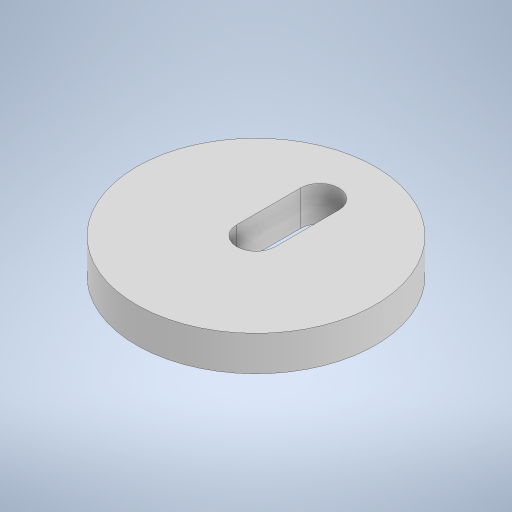
# Autodesk Inventor part: M3_15_ホーン
Saved by Autodesk Inventor 2024.1 (Build 281209000, 209)
## iProperties
Created: 2024-04-01
Part Number: M3_15_ホーン
Material: 一般
Document SubType Name: Modeling
Designer: hibik
Density: 1 g/cm^3
Appearance: 既定
Author: hibik
Autodesk Inventor part; units mm, degrees
ref_plane "YZ Plane" through (0, 0, 0) normal (1, 0, 0) x (0, 1, 0)
ref_plane "XZ Plane" through (0, 0, 0) normal (0, 1, 0) x (-1, 0, 0)
ref_plane "XY Plane" through (0, 0, 0) normal (0, 0, 1) x (1, 0, 0)
sketch "スケッチ1" plane through (0, 0, 0) normal (0, 1, 0) x (-1, 0, 0)
  circle A0 centre (0, 0) radius 22.5 construction
  circle A1 centre (0, 0) radius 25.5 construction
  line L0 (25.5, 1.2181) -> (25.5, -1.2181)
  line L1 (25.5, 1.2181) -> (22.3764, 2.355)
  line L2 (25.5, -1.2181) -> (22.3764, -2.355)
  line L3 (35.7, 0) -> (-35.7, 0) projected
  circle A2 centre (0, 0) radius 18.75
  line L4 (22.3764, -2.355) -> (18.647, -1.9625)
  line L5 (22.3764, 2.355) -> (18.647, 1.9625)
  line L6 (19.484, 11.2527) -> (16.2367, 9.3773)
  line L7 (22.8, 11.4846) -> (19.484, 11.2527)
  line L8 (22.8, 11.4846) -> (23.7909, 9.259)
  line L9 (23.7909, 9.259) -> (21.3997, 6.9499)
  line L10 (21.3997, 6.9499) -> (17.8331, 5.7916)
  line L11 (13.2226, 18.2047) -> (11.0189, 15.1706)
  line L12 (16.1576, 19.7653) -> (13.2226, 18.2047)
  line L13 (16.1576, 19.7653) -> (17.9681, 18.1351)
  line L14 (17.9681, 18.1351) -> (16.7229, 15.0531)
  line L15 (16.7229, 15.0531) -> (13.9357, 12.5443)
  line L16 (4.675, 22.009) -> (3.8958, 18.3408)
  line L17 (6.7214, 24.6284) -> (4.675, 22.009)
  line L18 (6.7214, 24.6284) -> (9.0384, 23.8755)
  line L19 (9.0384, 23.8755) -> (9.1544, 20.5535)
  line L20 (9.1544, 20.5535) -> (7.6287, 17.1279)
  line L21 (-4.6811, 22.0077) -> (-3.9009, 18.3397)
  line L22 (-3.8769, 25.233) -> (-4.6811, 22.0077)
  line L23 (-3.8769, 25.233) -> (-1.454, 25.4876)
  line L24 (-1.454, 25.4876) -> (0.0031, 22.5)
  line L25 (0.0031, 22.5) -> (0.0026, 18.75)
  line L26 (-13.2277, 18.201) -> (-11.0231, 15.1675)
  line L27 (-13.8049, 21.4746) -> (-13.2277, 18.201)
  line L28 (-13.8049, 21.4746) -> (-11.6951, 22.6927)
  line L29 (-11.6951, 22.6927) -> (-9.1487, 20.556)
  line L30 (-9.1487, 20.556) -> (-7.6239, 17.13)
  line L31 (-19.4871, 11.2473) -> (-16.2393, 9.3727)
  line L32 (-21.3459, 14.0031) -> (-19.4871, 11.2473)
  line L33 (-21.3459, 14.0031) -> (-19.9139, 15.974)
  line L34 (-19.9139, 15.974) -> (-16.7187, 15.0578)
  line L35 (-16.7187, 15.0578) -> (-13.9322, 12.5481)
  line L36 (-22.3771, 2.3488) -> (-18.6476, 1.9573)
  line L37 (-25.196, 4.1103) -> (-22.3771, 2.3488)
  line L38 (-25.196, 4.1103) -> (-24.6895, 6.4932)
  line L39 (-24.6895, 6.4932) -> (-21.3978, 6.9559)
  line L40 (-21.3978, 6.9559) -> (-17.8315, 5.7965)
  line L41 (-21.3978, -6.9559) -> (-17.8315, -5.7965)
  line L42 (-24.6895, -6.4932) -> (-21.3978, -6.9559)
  line L43 (-24.6895, -6.4932) -> (-25.196, -4.1103)
  line L44 (-25.196, -4.1103) -> (-22.3771, -2.3488)
  line L45 (-22.3771, -2.3488) -> (-18.6476, -1.9573)
  line L46 (-16.7187, -15.0578) -> (-13.9322, -12.5481)
  line L47 (-19.9139, -15.974) -> (-16.7187, -15.0578)
  line L48 (-19.9139, -15.974) -> (-21.3459, -14.0031)
  line L49 (-21.3459, -14.0031) -> (-19.4871, -11.2473)
  line L50 (-19.4871, -11.2473) -> (-16.2393, -9.3727)
  line L51 (-9.1487, -20.556) -> (-7.6239, -17.13)
  line L52 (-11.6951, -22.6927) -> (-9.1487, -20.556)
  line L53 (-11.6951, -22.6927) -> (-13.8049, -21.4746)
  line L54 (-13.8049, -21.4746) -> (-13.2277, -18.201)
  line L55 (-13.2277, -18.201) -> (-11.0231, -15.1675)
  line L56 (0.0031, -22.5) -> (0.0026, -18.75)
  line L57 (-1.454, -25.4876) -> (0.0031, -22.5)
  line L58 (-1.454, -25.4876) -> (-3.8769, -25.233)
  line L59 (-3.8769, -25.233) -> (-4.6811, -22.0077)
  line L60 (-4.6811, -22.0077) -> (-3.9009, -18.3397)
  line L61 (9.1544, -20.5535) -> (7.6287, -17.1279)
  line L62 (9.0384, -23.8755) -> (9.1544, -20.5535)
  line L63 (9.0384, -23.8755) -> (6.7214, -24.6284)
  line L64 (6.7214, -24.6284) -> (4.675, -22.009)
  line L65 (4.675, -22.009) -> (3.8958, -18.3408)
  line L66 (16.7229, -15.0531) -> (13.9357, -12.5443)
  line L67 (17.9681, -18.1351) -> (16.7229, -15.0531)
  line L68 (17.9681, -18.1351) -> (16.1576, -19.7653)
  line L69 (16.1576, -19.7653) -> (13.2226, -18.2047)
  line L70 (13.2226, -18.2047) -> (11.0189, -15.1706)
  line L71 (21.3997, -6.9499) -> (17.8331, -5.7916)
  line L72 (23.7909, -9.259) -> (21.3997, -6.9499)
  line L73 (23.7909, -9.259) -> (22.8, -11.4846)
  line L74 (22.8, -11.4846) -> (19.484, -11.2527)
  line L75 (19.484, -11.2527) -> (16.2367, -9.3773)
  circle A3 centre (0, 0) radius 11
  point P0 (25.5, 0)
  point P1 (23.2954, 10.3718)
  point P2 (17.0628, 18.9502)
  point P3 (7.8799, 24.2519)
  point P4 (-2.6655, 25.3603)
  point P5 (-12.75, 22.0836)
  point P6 (-20.6299, 14.9885)
  point P7 (-24.9428, 5.3017)
  point P8 (-24.9428, -5.3017)
  point P9 (-20.6299, -14.9885)
  point P10 (-12.75, -22.0836)
  point P11 (-2.6655, -25.3603)
  point P12 (7.8799, -24.2519)
  point P13 (17.0628, -18.9502)
  point P14 (23.2954, -10.3718)
  point P15 (17.8331, 5.7916)
  point P16 (16.2367, 9.3773)
  point P17 (13.9357, 12.5443)
  point P18 (11.0189, 15.1706)
  point P19 (7.6287, 17.1279)
  point P20 (3.8958, 18.3408)
  point P21 (0.0026, 18.75)
  point P22 (-3.9009, 18.3397)
  point P23 (-7.6239, 17.13)
  point P24 (-11.0231, 15.1675)
  point P25 (-13.9322, 12.5481)
  point P26 (-16.2393, 9.3727)
  point P27 (-17.8315, 5.7965)
  point P28 (-18.6476, 1.9573)
  point P29 (-18.6476, -1.9573)
  point P30 (-17.8315, -5.7965)
  point P31 (-16.2393, -9.3727)
  point P32 (-13.9322, -12.5481)
  point P33 (-11.0231, -15.1675)
  point P34 (-7.6239, -17.13)
  point P35 (-3.9009, -18.3397)
  point P36 (0.0026, -18.75)
  point P37 (3.8958, -18.3408)
  point P38 (7.6287, -17.1279)
  point P39 (11.0189, -15.1706)
  point P40 (13.9357, -12.5443)
  point P41 (16.2367, -9.3773)
  point P42 (17.8331, -5.7916)
  dimension "d5" = 37.5
  dimension "d0" = 45
  dimension "d1" = 51
  dimension "d3" = 20
  dimension "d4" = 20
  dimension "d14" = 4.71
  dimension "d18" = 360
  dimension "d23" = 22
  constraints: 150 end point, 31 point on line, 6 coincident, 3 centre point, 2 point on circle, 1 midpoint, 1 tangent, 1 vertical, 198 other
  measures "d0" diameter of A0
  measures "d1" diameter of A1
  measures "d3" angle of L3 L1
  measures "d4" angle of L3 L2
  measures "d14" distance of L2.end L1.end
  measures "d23" diameter of A3
extrude "押し出し1" add sketch "スケッチ1" along normal blind 5.5 contours A2 L3 A3 | L3 A3 A2 | A3 L3 | L3 A3
sketch "スケッチ2" plane through (0, 5.5, 0) normal (0, 1, 0) x (1, 0, 0)
  circle A0 centre (0, 10) radius 3
  circle A1 centre (0, 0) radius 3
  line L0 (-3, 10) -> (-3, 0)
  line L1 (3, 10) -> (3, 0)
  dimension "d30" = 6
  dimension "d31" = 6
  dimension "d32" = 10
  constraints: 4 end point, 4 point on circle, 2 centre point, 2 tangent, 1 coincident, 1 parallel, 1 vertical
  measures "d30" diameter of A0
  measures "d31" diameter of A1
  measures "d32" distance of point (0, 0) A0.centre
extrude "押し出し2" cut sketch "スケッチ2" against normal through all
